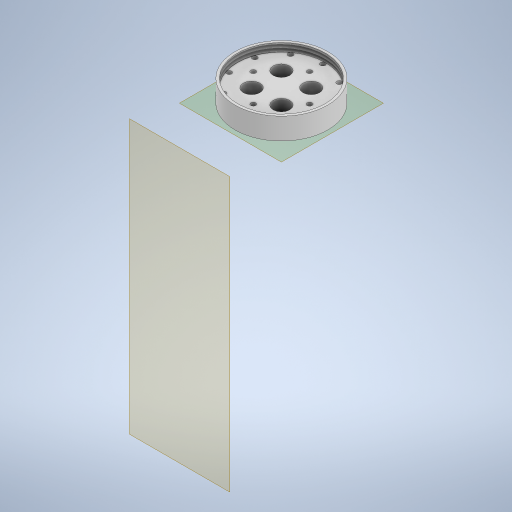
# Autodesk Inventor part: case v0 top
Saved by Autodesk Inventor 2023 (Build 270158000, 158)
## iProperties
Created: 2022-07-03
Part Number: case v0 top
Material: Generic
Document SubType Name: Modeling
Designer: Administrator
Density: 1 g/cm^3
Appearance: Default
Title: case v1
Author: Administrator
Autodesk Inventor part; units mm, degrees
ref_plane "YZ Plane" through (0, 0, 0) normal (1, 0, 0) x (0, 1, 0)
ref_plane "XZ Plane" through (0, 0, 0) normal (0, 1, 0) x (-1, 0, 0)
ref_plane "XY Plane" through (0, 0, 0) normal (0, 0, 1) x (1, 0, 0)
sketch "Sketch1" plane through (0, 0, 0) normal (0, 0, 1) x (1, 0, 0)
  line L0 (-27.5, 79) -> (27.5, 79)
  line L1 (27.5, 79) -> (27.5, -79)
  line L2 (27.5, -79) -> (-27.5, -79)
  line L3 (-27.5, -79) -> (-27.5, 79)
  line L4 (-20, 71.5) -> (20, 71.5)
  line L5 (20, 71.5) -> (20, -71.5)
  line L6 (20, -71.5) -> (-20, -71.5)
  line L7 (-20, -71.5) -> (-20, 71.5)
  point P0 (0, 0)
  point P1 (0, -79)
  dimension "d0" = 55
  dimension "d1" = 158
  dimension "d2" = 79
  dimension "d3" = 27.5
  dimension "d4" = 143
  dimension "d5" = 40
  dimension "d6" = 20
  dimension "d7" = 71.5
  constraints: 16 end point, 4 parallel, 2 horizontal, 2 perpendicular, 1 midpoint
  measures "d0" distance of L1.end L2.end
  measures "d1" distance of L0.end L1.end
  measures "d2" distance of point (0, -79) point (0, 0)
  measures "d3" distance from line of L3 point (0, 0)
  measures "d4" distance of L6.end L4.start
  measures "d5" distance of L5.end L6.end
  measures "d6" distance from line of L7 point (0, 0)
  measures "d7" distance from line of L4 point (0, 0)
extrude "Extrusion1" add sketch "Sketch1" along normal mid plane 3
sketch "Sketch2" plane through (-27.5, 79, -1.5) normal (0, 1, 0) x (1, 0, 0)
  circle A0 centre (27.5, -1.5) radius 28
  point P0 (27.5, -1.5)
  dimension "d10" = 56
  constraints: 1 centre point, 1 coincident
  measures "d10" diameter of A0
extrude "Extrusion2" add sketch "Sketch2" against normal blind 8
sketch "Sketch3" plane through (0, 0, 1.5) normal (0, 0, 1) x (1, 0, 0)
  line L0 (-25, 71) -> (25, 71)
  line L1 (25, 71) -> (25, -9)
  line L2 (25, -9) -> (-25, -9)
  line L3 (-25, -9) -> (-25, 71)
  circle A0 centre (-22, -6) radius 1.5
  circle A1 centre (-22, 68) radius 1.5
  circle A2 centre (22, -6) radius 1.5
  circle A3 centre (22, 68) radius 1.5
  line L4 (-28, 71) -> (28, 71) projected
  point P0 (0, 0)
  dimension "d13" = 80
  dimension "d14" = 50
  dimension "d15" = 25
  dimension "d16" = 3
  dimension "d18" = 3
  dimension "d19" = 3
  dimension "d20" = 3
  dimension "d21" = 44
  dimension "d22" = 44
  dimension "d23" = 22
  dimension "d24" = 22
  dimension "d25" = 74
  dimension "d27" = 74
  dimension "d77" = 0
  dimension "d78" = 3
  dimension "d79" = 3
  constraints: 8 end point, 4 centre point, 2 parallel, 1 horizontal, 1 perpendicular
  measures "d13" distance of L0.end L1.end
  measures "d14" distance of L1.end L2.end
  measures "d15" distance from line of L1 point (0, 0)
  measures "d16" diameter of A0
  measures "d18" diameter of A1
  measures "d19" diameter of A2
  measures "d20" diameter of A3
  measures "d21" distance of A2.centre A0.centre
  measures "d22" distance of A3.centre A1.centre
  measures "d23" horizontal distance of point (0, 0) A1.centre
  measures "d24" horizontal distance of point (0, 0) A0.centre
  measures "d25" distance of A0.centre A1.centre
  measures "d27" distance of A2.centre A3.centre
  measures "d77" distance between parallel lines of L4 L0
  measures "d78" distance from line of L0 A1.centre
  measures "d79" distance from line of L4 A3.centre
extrude "Extrusion3" cut sketch "Sketch3" against normal blind 6 contours A0 | A1 | A2 | A3
sketch "Sketch4" plane through (-27.5, -79, 1.5) normal (0, -1, 0) x (1, 0, 0)
  circle A0 centre (27.5, -1.5) radius 28
  point P0 (27.5, -1.5)
  constraints: 1 centre point, 1 coincident
extrude "Extrusion4" add sketch "Sketch4" along normal blind 8
sketch "Sketch5" plane through (0, 0, 0) normal (1, 0, 0) x (0, 1, 0)
  circle A0 centre (-81.5, 0) radius 1.5
  line L0 (-79, 28) -> (-79, -28) projected
  point P0 (0, 0)
  dimension "d33" = 3
  dimension "d34" = 2.5
  constraints: 1 centre point
  measures "d33" diameter of A0
  measures "d34" distance from line of A0.centre L0
extrude "Extrusion5" cut sketch "Sketch5" along normal through all both and the other way through all
thread "Thread1" size "M3x0.5" class "6H" standard "ANSI Metric M Profile" full length
sketch "Sketch6" plane through (0, -87, 0) normal (0, -1, 0) x (1, 0, 0)
  circle A0 centre (0, 0) radius 25
  circle A1 centre (0, 0) radius 22.5
  point P0 (0, 0)
  dimension "d39" = 50
  dimension "d40" = 45
  constraints: 2 centre point, 2 coincident
  measures "d39" diameter of A0
  measures "d40" diameter of A1
extrude "Extrusion6" add sketch "Sketch6" along normal blind 5
thread "Thread2" size "M50x2" class "6g" standard "ANSI Metric M Profile" full length
sketch "Sketch7" plane through (0, -79, 0) normal (0, 1, 0) x (1, 0, 0)
  circle A0 centre (0, 0) radius 22.5 projected
  line L0 (14.7394, 17) -> (-15.2606, 17)
  line L1 (-15.2606, 17) -> (-15.2606, 8)
  line L2 (-15.2606, 8) -> (14.7394, 8)
  line L3 (14.7394, 8) -> (14.7394, 17)
  line L4 (14.7394, -7.5337) -> (-15.2606, -7.5337)
  line L5 (-15.2606, -7.5337) -> (-15.2606, -16.5337)
  line L6 (-15.2606, -16.5337) -> (14.7394, -16.5337)
  line L7 (14.7394, -16.5337) -> (14.7394, -7.5337)
  point P0 (0, 0)
  point P1 (-14.7394, 17)
  point P2 (-15.2606, 16.5337)
  dimension "d45" = 9
  dimension "d46" = 9
  dimension "d47" = 30
  dimension "d48" = 8
  constraints: 16 end point, 4 parallel, 2 horizontal, 2 perpendicular, 2 point on circle, 2 point on line
  measures "d45" distance of L0.end L1.end
  measures "d46" distance of L4.end L5.end
  measures "d47" distance of L5.end L6.end
  measures "d48" distance from line of L2 point (0, 0)
extrude "Extrusion7" cut sketch "Sketch7" against normal blind 10 contours L5 L4 L7 L6 | L3 L2 L1 A0 L0
sketch "Sketch8" plane through (0, 79, 0) normal (0, 1, 0) x (1, 0, 0)
  circle A0 centre (0, -17) radius 1.5
  circle A1 centre (-17, 0) radius 1.5
  circle A2 centre (0, 17) radius 1.5
  circle A3 centre (17, 0) radius 1.5
  point P0 (0, 0)
  dimension "d51" = 3
  dimension "d52" = 3
  dimension "d53" = 3
  dimension "d54" = 3
  dimension "d55" = 34
  dimension "d56" = 34
  dimension "d57" = 17
  dimension "d58" = 17
  constraints: 4 centre point
  measures "d51" diameter of A0
  measures "d52" diameter of A1
  measures "d53" diameter of A2
  measures "d54" diameter of A3
  measures "d55" distance of A2.centre A0.centre
  measures "d56" distance of A1.centre A3.centre
  measures "d57" distance of A3.centre point (0, 0)
  measures "d58" distance of A2.centre point (0, 0)
extrude "Extrusion8" cut sketch "Sketch8" against normal blind 10
sketch "Sketch10" plane through (0, 79, 0) normal (0, 1, 0) x (1, 0, 0)
  circle A0 centre (0, 0) radius 28
  circle A1 centre (0, 0) radius 26.5
  point P0 (0, 0)
  dimension "d80" = 53
  dimension "d81" = 56
  constraints: 2 centre point, 2 coincident
  measures "d80" diameter of A1
  measures "d81" diameter of A0
extrude "Extrusion10" add sketch "Sketch10" along normal blind 5
thread "Thread3" size "M55x2" class "6H" standard "ANSI Metric M Profile" full length
sketch "Sketch11" plane through (0, 79, 0) normal (0, 1, 0) x (1, 0, 0)
  circle A0 centre (0, 0) radius 25 projected
  circle A1 centre (0, 25) radius 1.5
  point P0 (0, 0)
  dimension "d86" = 3
  constraints: 1 centre point, 1 vertical alignment, 1 other
  measures "d86" diameter of A1
extrude "Extrusion11" cut sketch "Sketch11" against normal up to surface (8 mm away) contours A1 A0 | A0 A1 picked at (-0.0591, 24.5002) picked at (0.0534, 25.4938)
pattern_circular "Circular Pattern1" count 10 over 360 about axis through (0, 79, 0) along (0, -1, 0) of "Extrusion11"
sketch "Sketch12" plane through (0, 0, -1.5) normal (0, 0, -1) x (-1, 0, 0)
  circle A0 centre (-22, -89.4052) radius 1.5
  point P0 (0, 0)
  dimension "d93" = 3
  dimension "d94" = 22
  constraints: 1 centre point
  measures "d93" diameter of A0
  measures "d94" horizontal distance of point (0, 0) A0.centre
extrude "Extrusion12" cut sketch "Sketch12" against normal blind 10
pattern_linear "Rectangular Pattern1" count 2 spacing 100 along (0, -1, 0) of "Extrusion3"
sketch "Sketch13" plane through (0, 79, -25) normal (0, 1, 0) x (1, 0, 0)
  circle A0 centre (9, -34) radius 5
  line L0 (14.7394, -17) -> (-15.2606, -17) projected
  circle A1 centre (9, -16) radius 5
  circle A2 centre (-9, -16) radius 5
  circle A3 centre (-9, -34) radius 5
  point P0 (0, -25)
  dimension "d100" = 10
  dimension "d101" = 10
  dimension "d104" = 18
  dimension "d108" = 9
  dimension "d109" = 9
  dimension "d110" = 9
  dimension "d111" = 10
  dimension "d112" = 10
  dimension "d113" = 9
  dimension "d114" = 9
  dimension "d115" = 9
  dimension "d116" = 9
  constraints: 4 centre point
  measures "d100" diameter of A0
  measures "d101" diameter of A1
  measures "d104" distance of A0.centre A1.centre
  measures "d108" horizontal distance of point (0, -25) A0.centre
  measures "d109" horizontal distance of point (0, -25) A0.centre
  measures "d110" horizontal distance of point (0, -25) A1.centre
  measures "d111" diameter of A2
  measures "d112" diameter of A3
  measures "d113" horizontal distance of point (0, -25) A2.centre
  measures "d114" horizontal distance of A3.centre point (0, -25)
  measures "d115" horizontal distance of point (0, -25) A2.centre
  measures "d116" horizontal distance of point (0, -25) A3.centre
extrude "Extrusion13" cut sketch "Sketch13" against normal up to surface (8 mm away)
sketch "Sketch14" plane through (-20, -71.5, 1.5) normal (0, 1, 0) x (1, 0, 0)
  arc A0 (4.7394, 18.0337) -> (4.7394, -15.0337) centre (20, 1.5) ccw projected
  line L0 (-7.5, 0) -> (47.5, 0) projected
  line L1 (-2.4455, 3.065) -> (42.5703, 3.065)
  line L2 (42.5703, 3.065) -> (42.5703, 0)
  line L3 (42.5703, 0) -> (-2.4455, 0)
  line L4 (-2.4455, 0) -> (-2.4455, 3.065)
  point P0 (20, 1.5)
  point P1 (-2.4455, 0)
  constraints: 8 end point, 2 parallel, 1 horizontal, 1 perpendicular, 1 point on circle, 1 point on line
extrude "Extrusion14" add sketch "Sketch14" along normal up to surface (142.5 mm away) contours L1 L2 L0 L4
ref_plane "Work Plane1" through (0, 0, 61.5) normal (0, 0, 1) x (1, 0, 0)
sketch "Sketch15" plane through (0, 0, 61.5) normal (0, 0, 1) x (1, 0, 0)
  line L0 (-22.4455, 66.5677) -> (-22.4455, -4.5677) projected
  line L1 (-22.4455, 66.5) -> (20.5545, 66.5)
  line L2 (20.5545, 66.5) -> (20.5545, -66.5)
  line L3 (20.5545, -66.5) -> (-22.4455, -66.5)
  line L4 (-22.4455, -66.5) -> (-22.4455, 66.5)
  line L5 (-22.4455, 56.5) -> (20.5545, 56.5)
  line L6 (-22.4455, 46.5) -> (20.5545, 46.5)
  line L7 (-22.4455, 36.5) -> (20.5545, 36.5)
  line L8 (-22.4455, 26.5) -> (20.5545, 26.5)
  line L9 (-22.4455, 16.5) -> (20.5545, 16.5)
  line L10 (-22.4455, 6.5) -> (20.5545, 6.5)
  line L11 (-22.4455, -3.5) -> (20.5545, -3.5)
  line L12 (-22.4455, -13.5) -> (20.5545, -13.5)
  line L13 (-22.4455, -23.5) -> (20.5545, -23.5)
  line L14 (-22.4455, -33.5) -> (20.5545, -33.5)
  line L15 (-22.4455, -43.5) -> (20.5545, -43.5)
  line L16 (-22.4455, -53.5) -> (20.5545, -53.5)
  line L17 (-22.4455, -63.5) -> (20.5545, -63.5)
  line L18 (15.5545, 66.5) -> (15.5545, -66.5)
  line L19 (10.5545, 66.5) -> (10.5545, -66.5)
  line L20 (5.5545, 66.5) -> (5.5545, -66.5)
  line L21 (0.5545, 66.5) -> (0.5545, -66.5)
  line L22 (-4.4455, 66.5) -> (-4.4455, -66.5)
  line L23 (-9.4455, 66.5) -> (-9.4455, -66.5)
  line L24 (-14.4455, 66.5) -> (-14.4455, -66.5)
  line L25 (-19.4455, 66.5) -> (-19.4455, -66.5)
  line L26 (-24.4455, 66.5) -> (-24.4455, -66.5)
  point P0 (0, 0)
  point P1 (15.5545, -43.5)
  point P2 (15.5545, -53.5)
  point P3 (5.5545, -43.5)
  point P4 (5.5545, -53.5)
  point P5 (10.5545, -53.5)
  point P6 (10.5545, -43.5)
  point P7 (-4.4455, -43.5)
  point P8 (-4.4455, -53.5)
  point P9 (0.5545, -53.5)
  point P10 (0.5545, -43.5)
  point P11 (-14.4455, -43.5)
  point P12 (-14.4455, -53.5)
  point P13 (-9.4455, -53.5)
  point P14 (-9.4455, -43.5)
  point P15 (-19.4455, -53.5)
  point P16 (-19.4455, -43.5)
  point P17 (10.5545, -23.5)
  point P18 (10.5545, -33.5)
  point P19 (15.5545, -33.5)
  point P20 (15.5545, -23.5)
  point P21 (0.5545, -23.5)
  point P22 (0.5545, -33.5)
  point P23 (5.5545, -33.5)
  point P24 (5.5545, -23.5)
  point P25 (-9.4455, -23.5)
  point P26 (-9.4455, -33.5)
  point P27 (-4.4455, -33.5)
  point P28 (-4.4455, -23.5)
  point P29 (-19.4455, -23.5)
  point P30 (-19.4455, -33.5)
  point P31 (-14.4455, -33.5)
  point P32 (-14.4455, -23.5)
  point P33 (15.5545, -3.5)
  point P34 (15.5545, -13.5)
  point P35 (5.5545, -3.5)
  point P36 (5.5545, -13.5)
  point P37 (10.5545, -13.5)
  point P38 (10.5545, -3.5)
  point P39 (-4.4455, -3.5)
  point P40 (-4.4455, -13.5)
  point P41 (0.5545, -13.5)
  point P42 (0.5545, -3.5)
  point P43 (-14.4455, -3.5)
  point P44 (-14.4455, -13.5)
  point P45 (-9.4455, -13.5)
  point P46 (-9.4455, -3.5)
  point P47 (-19.4455, -13.5)
  point P48 (-19.4455, -3.5)
  point P49 (-22.4455, -4.5677)
  point P50 (15.5545, 16.5)
  point P51 (15.5545, 6.5)
  point P52 (5.5545, 16.5)
  point P53 (5.5545, 6.5)
  point P54 (10.5545, 6.5)
  point P55 (10.5545, 16.5)
  point P56 (-4.4455, 16.5)
  point P57 (-4.4455, 6.5)
  point P58 (0.5545, 6.5)
  point P59 (0.5545, 16.5)
  point P60 (-14.4455, 16.5)
  point P61 (-14.4455, 6.5)
  point P62 (-9.4455, 6.5)
  point P63 (-9.4455, 16.5)
  point P64 (-19.4455, 6.5)
  point P65 (-19.4455, 16.5)
  point P66 (-19.4455, 36.5)
  point P67 (-19.4455, 26.5)
  point P68 (-14.4455, 26.5)
  point P69 (-14.4455, 36.5)
  point P70 (-19.4455, 56.5)
  point P71 (-19.4455, 46.5)
  point P72 (-14.4455, 46.5)
  point P73 (-14.4455, 56.5)
  point P74 (-9.4455, 56.5)
  point P75 (-9.4455, 46.5)
  point P76 (-4.4455, 46.5)
  point P77 (-4.4455, 56.5)
  point P78 (-9.4455, 36.5)
  point P79 (-9.4455, 26.5)
  point P80 (-4.4455, 26.5)
  point P81 (-4.4455, 36.5)
  point P82 (10.5545, 36.5)
  point P83 (10.5545, 26.5)
  point P84 (15.5545, 26.5)
  point P85 (15.5545, 36.5)
  point P86 (10.5545, 56.5)
  point P87 (10.5545, 46.5)
  point P88 (15.5545, 46.5)
  point P89 (15.5545, 56.5)
  point P90 (0.5545, 56.5)
  point P91 (0.5545, 46.5)
  point P92 (5.5545, 46.5)
  point P93 (5.5545, 56.5)
  point P94 (0.5545, 36.5)
  point P95 (0.5545, 26.5)
  point P96 (5.5545, 26.5)
  point P97 (5.5545, 36.5)
  dimension "d122" = 43
  dimension "d123" = 133
  dimension "d124" = 66.5
  dimension "d127" = 10
  dimension "d134" = 5
  constraints: 52 end point, 2 horizontal, 2 parallel, 1 perpendicular, 1 point on line, 1 vertical, 66 other
  measures "d122" distance of L1.start L1.end
  measures "d123" distance of L3.end L1.start
  measures "d124" distance from line of point (0, 0) L1
  measures "d127" distance of L1.start L5.start
  measures "d134" distance of L1.end L18.start
extrude "Extrusion15" cut sketch "Sketch15" against normal up to surface (63.065 mm away) contours L5 L24 L6 L25 | L7 L24 L8 L25 | L5 L22 L6 L23 | L9 L25 L10 L0 | L7 L22 L8 L23 | L5 L20 L6 L21 | L11 L25 L12 L4 L0 | L9 L23 L10 L24 | L7 L20 L8 L21 | L5 L18 L6 L19 | L11 L23 L12 L24 | L9 L21 L10 L22 | L13 L24 L14 L25 | L7 L18 L8 L19 | L11 L21 L12 L22 | L9 L19 L10 L20 | L15 L25 L16 L4 | L13 L22 L14 L23 | L11 L19 L12 L20 | L15 L23 L16 L24 | L9 L2 L10 L18 | L13 L20 L14 L21 | L11 L2 L12 L18 | L15 L21 L16 L22 | L13 L18 L14 L19 | L15 L19 L16 L20 | L15 L2 L16 L18
ref_plane "Work Plane2" through (0, 71, 0) normal (0, -1, 0) x (1, 0, 0)
split "Split1" plane through (0, 71, 0) removes the side toward (0, -1, 0)
sketch "Sketch16" plane through (0, 71, 0) normal (0, -1, 0) x (1, 0, 0)
  line L0 (-18.7383, 20.8597) -> (-20.8596, 18.7383)
  line L1 (-20.8596, 18.7383) -> (18.7383, -20.8597)
  line L2 (18.7383, -20.8597) -> (20.8596, -18.7383)
  line L3 (20.8596, -18.7383) -> (-18.7383, 20.8597)
  point P0 (0, 0)
  point P1 (0, 28)
  dimension "d142" = 3
  dimension "d143" = 1.5
  dimension "d144" = 56
  dimension "d146" = 28
  constraints: 8 end point, 2 parallel, 1 perpendicular
  measures "d142" distance of L0.start L0.end
  measures "d143" distance from line of point (0, 0) L3
  measures "d144" distance of L2.end L0.start
  measures "d146" distance from line of L0 point (0, 0)
extrude "Extrusion16" cut sketch "Sketch16" against normal blind 5
body "Solid1"
